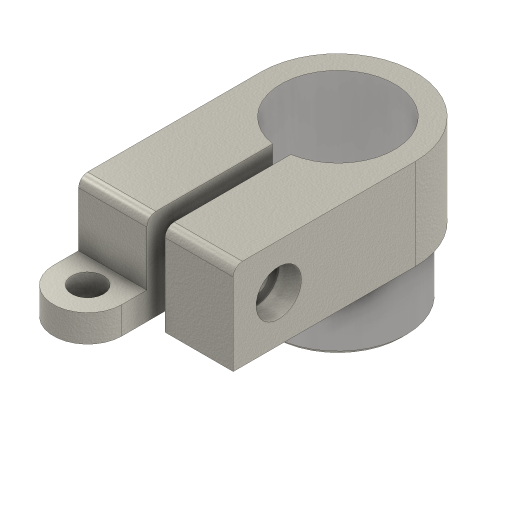
# Autodesk Inventor part: Part030. Notched attach
Saved by Autodesk Inventor 2023.2 (Build 272271030, 271C)
## iProperties
Created: 2023-10-11
Part Number: Part030. Notched attach
Material: Steel, Cast
Document SubType Name: Modeling
Designer: User
Mass: 1703.14 g
Surface Area: 473.85 cm^2
Volume: 216.96 cm^3
Density: 7.85 g/cm^3
Appearance: Steel - Cast
Author: User
Autodesk Inventor part; units mm, degrees
ref_plane "YZ Plane" through (0, 0, 0) normal (1, 0, 0) x (0, 1, 0)
ref_plane "XZ Plane" through (0, 0, 0) normal (0, 1, 0) x (-1, 0, 0)
ref_plane "XY Plane" through (0, 0, 0) normal (0, 0, 1) x (1, 0, 0)
sketch "Sketch1" plane through (0, 0, 0) normal (0, 1, 0) x (-1, 0, 0)
  line L0 (34, 91) -> (34, 0)
  arc A0 (-34, 0) -> (34, 0) centre (0, 0) ccw
  line L1 (-34, 0) -> (-34, 80)
  line L2 (-34, 80) -> (4, 80)
  line L3 (4, 80) -> (4, 91)
  arc A1 (34, 91) -> (4, 91) centre (19, 91) ccw
  dimension "d0" = 34
  dimension "d1" = 15
  dimension "d2" = 91
  dimension "d3" = 80
  constraints: 8 end point, 4 point on circle, 4 tangent, 2 centre point, 2 perpendicular, 1 coincident, 1 parallel, 1 vertical
  measures "d0" radius of A0
  measures "d1" radius of A1
  measures "d2" vertical distance of A1.centre point (0, 0)
  measures "d3" distance from line of L2 point (0, 0)
extrude "Extrusion1" add sketch "Sketch1" along normal blind 40
sketch "Sketch2" plane through (0, 40, 0) normal (0, 1, 0) x (1, 0, 0)
  line L0 (-4, -80) -> (34, -80) projected
  arc A0 (34, 0) -> (-34, 0) centre (0, 0) ccw projected
  line L1 (-4, -80) -> (4, -80)
  line L2 (4, -80) -> (4, 0)
  line L3 (4, 0) -> (-4, 0)
  line L4 (-4, 0) -> (-4, -80)
  dimension "d6" = 8
  constraints: 8 end point, 2 parallel, 1 horizontal, 1 midpoint, 1 perpendicular
  measures "d6" distance of L3.end L2.end
extrude "Extrusion2" cut sketch "Sketch2" against normal through all
sketch "Sketch3" plane through (-4, 0, 91) normal (1, 0, 0) x (0, 0, -1)
  line L0 (0, 40) -> (91, 40) projected
  line L1 (11, 0) -> (11, 40) projected
  line L2 (-15, 0) -> (-15, 40) projected
  line L3 (11, 40) -> (-15, 40)
  line L4 (-15, 40) -> (-15, 12)
  line L5 (-15, 12) -> (11, 12)
  line L6 (11, 12) -> (11, 40)
  line L7 (0, 0) -> (-15, 0) projected
  point P0 (11, 12)
  dimension "d9" = 12
  constraints: 8 end point, 2 parallel, 1 horizontal, 1 perpendicular, 1 point on line
  measures "d9" distance between parallel lines of L7 L5
extrude "Extrusion3" cut sketch "Sketch3" against normal through all
sketch "Sketch4" plane through (0, 0, 0) normal (0, -1, 0) x (1, 0, 0)
  line L0 (4, 80) -> (4, 0) projected
  line L1 (4, 0) -> (-4, 0) projected
  line L2 (-4, 91) -> (-4, 0) projected
  arc A0 (-34, 0) -> (34, 0) centre (0, 0) ccw projected
  circle A1 centre (0, 0) radius 30
  point P0 (-4, 29.7321)
  point P1 (4, 29.7321)
  dimension "d12" = 60
  constraints: 1 centre point, 1 coincident
  measures "d12" diameter of A1
extrude "Extrusion4" add sketch "Sketch4" along normal blind 30
chamfer "Chamfer1" distance 2 angle 45 1 edges at (-4, -30, -29.7321)
fillet "Fillet1" radius 4 2 edges at (-19, 40, 80) (19, 40, 80)
sketch "Sketch5" plane through (-4, 12, 91) normal (0, 1, 0) x (1, 0, 0)
  arc A0 (-30, 0) -> (0, 0) centre (-15, 0) ccw projected
  point P0 (4, 91)
  constraints: 1 coincident
hole "Hole1" at (-19, 12, 91) direction (0, -1, 0) diameter 14 end through all
sketch "Sketch6" plane through (0, -30, 0) normal (0, -1, 0) x (1, 0, 0)
  circle A0 centre (0, 0) radius 28 projected
  constraints: 1 coincident
hole "Hole2" at (0, -30, 0) direction (0, 1, 0) diameter 50 end through all
sketch "Sketch7" plane through (34, 0, 80) normal (1, 0, 0) x (0, 0, -1)
  line L0 (80, 0) -> (80, 40) projected
  line L1 (4, 40) -> (80, 40) projected
  point P0 (20, 20)
  dimension "d33" = 60
  dimension "d34" = 20
  measures "d33" distance from line of L0 point (20, 20)
  measures "d34" distance from line of point (20, 20) L1
hole "Hole3" at (34, 20, 60) direction (-1, 0, 0) diameter 12 end through all counterbore diameter 20 counterbore depth 10
body "Solid1"
